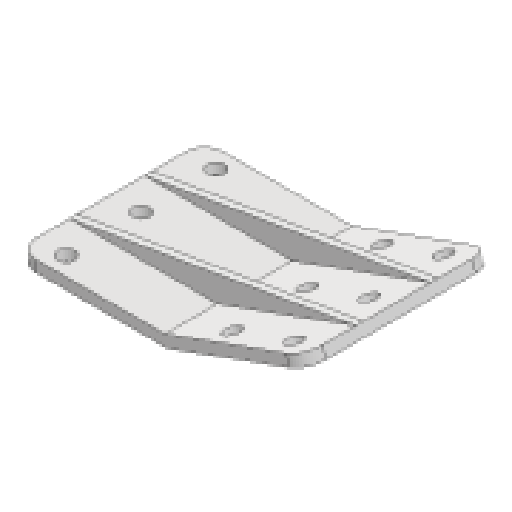
# Autodesk Inventor part: Angle
Saved by Autodesk Inventor 2024 (Build 280153000, 153)
## iProperties
Created: 2025-04-26
Part Number: Angle
Material: Generic
Document SubType Name: Modeling
Designer: Binara
Density: 1 g/cm^3
Appearance: Default
Author: Binara
## iProperties of the stored document Angle_3DPrint.ipt
Created: 2025-04-26
Part Number: Angle_3DPrint
Material: Generic
Document SubType Name: Modeling
Designer: Binara
Density: 1 g/cm^3
Appearance: Default
Author: Binara
Autodesk Inventor part; units mm, degrees
ref_plane "YZ Plane" through (0, 0, 0) normal (1, 0, 0) x (0, 1, 0)
ref_plane "XZ Plane" through (0, 0, 0) normal (0, 1, 0) x (-1, 0, 0)
sketch "Sketch1" plane through (0, 0, 0) normal (0, 0, 1) x (1, 0, 0)
  line L0 (0, 0) -> (-40, 0)
  line L1 (-40, 0) -> (-40, 3)
  line L2 (-40, 3) -> (0, 3)
  line L3 (0, 3) -> (0, 0)
  line L4 (0, 0) -> (-1.0261, 2.8191)
  line L5 (-1.0261, 2.8191) -> (36.5616, 16.4999)
  line L6 (36.5616, 16.4999) -> (37.5877, 13.6808)
  line L7 (37.5877, 13.6808) -> (0, 0)
  point P0 (-0.529, 3)
  dimension "d0" = 160
  dimension "d1" = 3
  dimension "d2" = 3
  dimension "d3" = 40
  dimension "d4" = 40
  constraints: 16 end point, 4 parallel, 2 perpendicular, 1 horizontal
  measures "d0" angle of L2 L5
  measures "d1" distance of L5.end L6.end
  measures "d2" distance of L0.end L1.end
  measures "d3" distance of L0.start L0.end
  measures "d4" distance of L6.end L0.start
extrude "Extrusion1" add sketch "Sketch1" along normal blind 50
sketch "Sketch2" plane through (-40, 3, 0) normal (0, 1, 0) x (1, 0, 0)
  line L0 (0, 0) -> (40, 0) projected
  line L1 (0, -50) -> (40, -50) projected
  circle A0 centre (8, -45) radius 2.25
  circle A1 centre (8, -25) radius 2.25
  circle A2 centre (8, -5) radius 2.25
  line L2 (8, 0) -> (8, -50)
  line L3 (0, 0) -> (0, -50) projected
  point P0 (8, -25)
  dimension "d7" = 4.5
  dimension "d8" = 4.5
  dimension "d9" = 4.5
  dimension "d10" = 20
  dimension "d12" = 8
  dimension "d13" = 20
  constraints: 4 point on line, 3 centre point, 2 end point, 1 midpoint, 1 perpendicular
  measures "d7" diameter of A0
  measures "d8" diameter of A1
  measures "d9" diameter of A2
  measures "d10" distance of A1.centre A2.centre
  measures "d12" distance between parallel lines of L3 L2
  measures "d13" distance of point (8, -25) A0.centre
extrude "Extrusion2" cut sketch "Sketch2" against normal blind 50 contours L2 A2 | A2 L2 | L2 A0 | A0 L2 | L2 A1 | A1 L2
ref_plane "Work Plane1" through (-0.529, 3, 0) normal (0.9848078, 0.1736482, 0) x (0, 0, -1)
mirror "Mirror1" about plane through (-0.529, 3, 0) normal (0.9848078, 0.1736482, 0) of "Extrusion2"
fillet "Fillet1" radius 5 4 edges at (37.0747, 15.0903, 0) (37.0747, 15.0903, 50) (-40, 1.5, 50) (-40, 1.5, 0)
sketch "Sketch3" plane through (-0.529, 3, 0) normal (0.9848078, 0.1736482, 0) x (0, 0, -1)
  line L0 (-5, 6.8541) -> (-45, 6.8541) projected
  ellipse E0 centre (-45, 5.4649) end of major axis (-47.25, 5.4649) minor radius 0.3907 projected
  ellipse E1 centre (-25, 5.4649) end of major axis (-27.25, 5.4649) minor radius 0.3907 projected
  ellipse E2 centre (-5, 5.4649) end of major axis (-7.25, 5.4649) minor radius 0.3907 projected
  line L1 (-25, 5.4649) -> (-25, 19.1248)
  line L2 (-45, 5.4649) -> (-25, 5.4649)
  line L3 (-36, -8.762) -> (-34, -8.762)
  line L4 (-34, -8.762) -> (-34, 19.6918)
  line L5 (-34, 19.6918) -> (-36, 19.6918)
  line L6 (-36, 19.6918) -> (-36, -8.762)
  line L7 (-36, -8.762) -> (-34, 19.6918) construction
  line L8 (-34, -8.762) -> (-36, 19.6918) construction
  ellipse E3 centre (-5, 5.9858) end of major axis (0, 5.9858) minor radius 0.8682 (0, 5.9858) -> (-5, 6.8541) ccw projected
  line L9 (-5, 6.8541) -> (-45, 6.8541) projected
  ellipse E4 centre (-45, 5.9858) end of major axis (-40, 5.9858) minor radius 0.8682 (-45, 6.8541) -> (-50, 5.9858) ccw projected
  line L10 (-50, 0) -> (-50, 5.9858) projected
  line L11 (0, 0) -> (-50, 0) projected
  line L12 (0, 0) -> (0, 5.9858) projected
  ellipse E5 centre (-45, 5.4649) end of major axis (-47.25, 5.4649) minor radius 0.3907 projected
  ellipse E6 centre (-25, 5.4649) end of major axis (-27.25, 5.4649) minor radius 0.3907 projected
  ellipse E7 centre (-5, 5.4649) end of major axis (-7.25, 5.4649) minor radius 0.3907 projected
  line L13 (-14, -8.762) -> (-16, -8.762)
  line L14 (-16, -8.762) -> (-16, 19.6918)
  line L15 (-16, 19.6918) -> (-14, 19.6918)
  line L16 (-14, 19.6918) -> (-14, -8.762)
  line L17 (-14, -8.762) -> (-16, 19.6918) construction
  line L18 (-16, -8.762) -> (-14, 19.6918) construction
  point P0 (0, -3.0463)
  point P1 (-35, 5.4649)
  point P2 (-15, 5.4649)
  point P3 (-14, 0)
  point P4 (-14, 6.8541)
  point P5 (-16, 6.8541)
  point P6 (-16, 0)
  point P7 (-36, 0)
  point P8 (-34, 0)
  point P9 (-34, 6.8541)
  point P10 (-36, 6.8541)
  dimension "d17" = 2
  constraints: 28 end point, 5 symmetric about line, 3 midpoint, 2 horizontal, 2 parallel, 1 perpendicular, 1 vertical, 8 other
  measures "d17" distance of L4.end L5.end
extrude "Extrusion3" add sketch "Sketch3" against normal up to next contours L16 L11 L14 L0 | L4 L2 L6 L0 | L11 L6 L2 L4
mirror "Mirror2" about plane through (-0.529, 3, 0) normal (0.9848078, 0.1736482, 0) of "Extrusion3"
sketch "Sketch4" plane through (-0.529, 3, 34) normal (-0.3420201, 0.9396926, 0) x (0.9396926, 0.3420201, 0)
  circle A0 centre (13.7993, 29) radius 2.25
  circle A1 centre (13.7993, 9) radius 2.25
  circle A2 centre (13.7993, -11) radius 2.25
  point P0 (-0.529, 34)
  constraints: 3 centre point
extrude "Extrusion4" cut sketch "Sketch4" against normal blind 10
equation "\"d13\" = d10"
body "Solid1"
